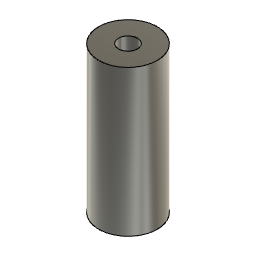
EC11 Coupler v1 (Autodesk Fusion 360 design; units mm, degrees)
Autodesk Fusion 360 part; units mm, degrees
cylinder "CylinderPrimitive1" add diameter 20 height 35 placed x (1, 0, 0) y (0, 1, 0) z (0, 0, 1) at (0, 0, 0)
hole "Hole1" at (0, 0, 35) direction (0, 0, -1) diameter 4.5 depth 15 tip angle 118
sketch "Sketch2" plane through (0, 0, 0) normal (0, 0, -1) x (1, 0, 0)
  circle A0 centre (0, 0) radius 10
  circle A1 centre (0, 0) radius 3
  line L0 (-3, -0.0031) -> (1.5, -0.0031)
  line L1 (1.5, -0.0031) -> (1.5, -2.5981)
  line L2 (1.5, -0.0031) -> (1.5, 2.5981)
  constraint coincident A0.centre A1.centre
  constraint coincident A1 L0.start
  constraint horizontal L0
  constraint coincident A1 L1.end
  constraint perpendicular L0 L1
  constraint coincident A1 L2.end
  constraint perpendicular L0 L2
extrude "Extrude1" cut sketch "Sketch2" against normal blind 21 contours A1 L0 L2 | A1 L0 L1
move_face "OffsetFaces1" offset -3 1 faces at (9.9503, -0.9957, 11.6667)
